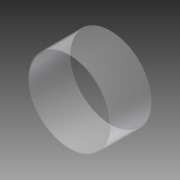
# Autodesk Inventor part: polycarb hopper walls
Saved by Autodesk Inventor 2012 (Build 160160000, 160)
## iProperties
Created: 2013-07-07
Part Number: polycarb hopper walls
Material: Default
Document SubType Name: Modeling
Designer: Bryce
Density: 1 g/cm^3
Author: Bryce
Autodesk Inventor part; units mm, degrees
ref_plane "YZ Plane" through (0, 0, 0) normal (1, 0, 0) x (0, 1, 0)
ref_plane "XZ Plane" through (0, 0, 0) normal (0, 1, 0) x (-1, 0, 0)
ref_plane "XY Plane" through (0, 0, 0) normal (0, 0, 1) x (1, 0, 0)
sketch "Sketch1" plane through (0, 0, 0) normal (0, 0, 1) x (1, 0, 0)
  circle A0 centre (0, 0) radius 152.4
  circle A1 centre (0, 0) radius 149.225
  dimension "d0" = 304.8
  dimension "d1" = 298.45
  constraints: 2 centre point, 2 coincident
  measures "d0" diameter of A0
  measures "d1" diameter of A1
extrude "Extrusion1" add sketch "Sketch1" along normal blind 152.4
body "Solid1"
